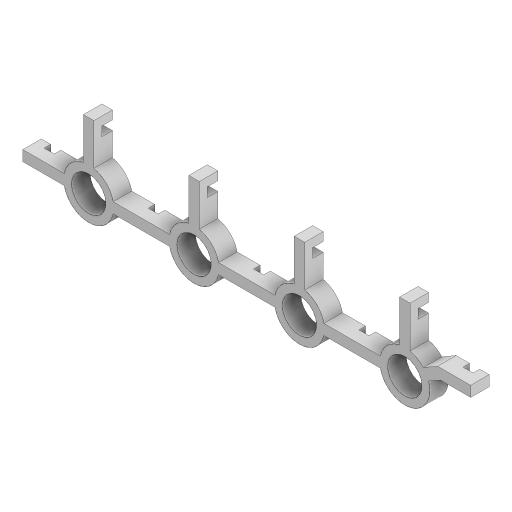
# Autodesk Inventor part: smic_jig_2
Saved by Autodesk Inventor 2024 (Build 280153000, 153)
## iProperties
Created: 2024-04-26
Part Number: smic_jig_2
Material: 一般
Document SubType Name: Modeling
Designer: TEA
Density: 1 g/cm^3
Appearance: 預設
Author: TEA
Autodesk Inventor part; units mm, degrees
ref_plane "YZ Plane" through (0, 0, 0) normal (1, 0, 0) x (0, 1, 0)
ref_plane "XZ Plane" through (0, 0, 0) normal (0, 1, 0) x (-1, 0, 0)
ref_plane "XY Plane" through (0, 0, 0) normal (0, 0, 1) x (1, 0, 0)
sketch "草圖1" plane through (0, 0, 0) normal (0, 0, 1) x (1, 0, 0)
  circle A0 centre (0, 0) radius 6.5
  circle A1 centre (0, 0) radius 9.5
  line L0 (0, 0) -> (16.7794, 0)
  circle A2 centre (40, 0) radius 6.5
  circle A3 centre (40, 0) radius 9.5
  circle A4 centre (80, 0) radius 6.5
  circle A5 centre (80, 0) radius 9.5
  circle A6 centre (120, 0) radius 6.5
  circle A7 centre (120, 0) radius 9.5
  line L1 (-25, 2) -> (128, 2)
  line L2 (128, 2) -> (128, -2)
  line L3 (128, -2) -> (-25, -2)
  line L4 (-25, -2) -> (-25, 2)
  line L5 (-2, 0) -> (2, 0)
  line L6 (2, 0) -> (2, 25)
  line L7 (2, 25) -> (-2, 25)
  line L8 (-2, 25) -> (-2, 0)
  line L9 (42, 0) -> (42, 25)
  line L10 (38, 0) -> (42, 0)
  line L11 (42, 25) -> (38, 25)
  line L12 (38, 25) -> (38, 0)
  line L13 (82, 0) -> (82, 25)
  line L14 (78, 0) -> (82, 0)
  line L15 (82, 25) -> (78, 25)
  line L16 (78, 25) -> (78, 0)
  line L17 (122, 0) -> (122, 25)
  line L18 (118, 0) -> (122, 0)
  line L19 (122, 25) -> (118, 25)
  line L20 (118, 25) -> (118, 0)
  line L21 (0, 0) -> (-12.3433, -7.1264)
  line L22 (0, 0) -> (14.2529, 0) construction
  line L23 (-12.4545, -9.5) -> (-25, -9.5)
  line L24 (-25, -9.5) -> (-25, -5.5)
  line L25 (-0.5359, 2) -> (14.2529, 2)
  line L26 (-12.4545, -9.5) -> (-7.0429, -6.3756)
  line L27 (0.5359, -2) -> (14.2529, -2)
  line L28 (-13.5263, -5.5) -> (-9.0429, -2.9115)
  line L29 (-25, -5.5) -> (-13.5263, -5.5)
  line L30 (-12.4545, 9.5) -> (-25, 9.5)
  line L31 (-25, 9.5) -> (-25, 5.5)
  line L32 (-12.4545, 9.5) -> (-7.0429, 6.3756)
  line L33 (-13.5263, 5.5) -> (-9.0429, 2.9115)
  line L34 (-25, 5.5) -> (-13.5263, 5.5)
  line L35 (42, 25) -> (78, 25)
  line L36 (60, 25) -> (60, 20)
  line L37 (132.4545, 9.5) -> (145, 9.5)
  line L38 (145, 9.5) -> (145, 5.5)
  line L39 (145, 5.5) -> (133.5263, 5.5)
  line L40 (133.5263, 5.5) -> (129.0429, 2.9115)
  line L41 (132.4545, 9.5) -> (127.0429, 6.3756)
  point P0 (-9.2871, -2)
  point P1 (-9.2871, 2)
  point P2 (30.7129, -2)
  point P3 (49.2871, -2)
  point P4 (70.7129, -2)
  point P5 (89.2871, -2)
  point P6 (110.7129, -2)
  point P7 (129.2871, -2)
  point P8 (129.2871, 2)
  point P9 (110.7129, 2)
  point P10 (89.2871, 2)
  point P11 (70.7129, 2)
  point P12 (49.2871, 2)
  point P13 (30.7129, 2)
  point P14 (9.2871, 2)
  point P15 (9.2871, -2)
  point P16 (118, 9.2871)
  point P17 (122, 9.2871)
  point P18 (78, 9.2871)
  point P19 (82, 9.2871)
  point P20 (38, 9.2871)
  point P21 (42, 9.2871)
  point P22 (-2, 9.2871)
  point P23 (2, 9.2871)
  point P24 (86.1847, -2)
  point P25 (113.8153, -2)
  point P26 (113.8153, 2)
  point P27 (86.1847, 2)
  point P28 (33.8153, -2)
  point P29 (33.8153, 2)
  point P30 (46.1847, -2)
  point P31 (73.8153, -2)
  point P32 (73.8153, 2)
  point P33 (46.1847, 2)
  point P34 (126.1847, 2)
  point P35 (126.1847, -2)
  dimension "d0" = 13
  dimension "d2" = 19
  dimension "d13" = 40
  dimension "d18" = 4
  dimension "d19" = 2
  dimension "d20" = 8
  dimension "d21" = 25
  dimension "d43" = 4
  dimension "d44" = 2
  dimension "d45" = 25
  dimension "d49" = 40
  dimension "d69" = 150
  dimension "d74" = 2
  dimension "d75" = 4
  dimension "d76" = 25
  dimension "d81" = 5
  constraints: 84 end point, 12 symmetric about line, 11 coincident, 8 centre point, 8 horizontal, 6 parallel, 5 midpoint, 3 perpendicular, 2 point on circle, 1 equal length, 1 tangent, 1 vertical, 45 other
  measures "d0" diameter of A0
  measures "d2" diameter of A1
  measures "d13" distance of A0.centre A2.centre
  measures "d18" distance of L1.end L2.end
  measures "d19" distance from line of point (0, 0) L1
  measures "d20" distance from line of A6.centre L2
  measures "d21" distance from line of point (0, 0) L4
  measures "d43" distance of L7.end L6.end
  measures "d44" distance from line of point (0, 0) L6
  measures "d45" distance of L7.end L5.start
  measures "d49" distance of L5.end L9.start
  measures "d69" angle of L21 L22
  measures "d74" distance between parallel lines of L21 L26
  measures "d75" distance of L23.end L24.end
  measures "d76" distance from line of A0.centre L24
  measures "d81" distance of L36.start L36.end
extrude "擠出1" add sketch "草圖1" along normal blind 7 contours L0 A1 L3 A0 | A0 L1 A1 L0 | A0 L6 A1 L1 | L3 A1 L21 A0 | A1 L1 A3 L3 | A0 L8 A1 L6 | L21 A1 L3 A0 | A0 L1 A1 L8 | A1 L8 L7 L6 | L3 A1 L1 A0 | L1 A2 L3 A3 | A3 L12 A2 L1 | L3 L4 L1 A1 | L3 A2 A3 | L12 L11 L9 A3 | A3 L9 A2 L12 | L3 A2 L1 A3 | A3 L1 A5 L3 | A3 L1 A2 L9 | L3 A4 A5 | A5 L1 A4 L3 | A5 L16 A4 L1 | L3 A4 L1 A5 | A5 L1 A7 L3 | L16 L15 L13 A5 | A5 L13 A4 L16 | L3 A6 L2 L1 L17 A7 | A7 L1 A6 L3 | A5 L1 A4 L13 | A7 L20 A6 L1 | L20 L19 L17 A7 | A7 L17 A6 L20 | A7 L41 L37 L38 L39 L40 | A6 L1 L2 L3
sketch "草圖3" plane through (49.2871, -2, 0) normal (0, -1, 0) x (1, 0, 0)
  line L0 (-31.1871, 0) -> (-27.3871, 0)
  line L1 (-27.3871, 0) -> (-27.3871, 2.5)
  line L2 (-27.3871, 2.5) -> (-31.1871, 2.5)
  line L3 (-31.1871, 2.5) -> (-31.1871, 0)
  line L4 (-31.1871, 0) -> (-27.3871, 2.5) construction
  line L5 (-27.3871, 0) -> (-31.1871, 2.5) construction
  line L6 (-18.5742, 0) -> (-18.5742, 7) projected
  line L7 (-40, 0) -> (-18.5742, 0) projected
  line L8 (-40, 0) -> (-18.5742, 0)
  line L9 (-29.2871, 0) -> (-29.2871, 1.25)
  line L10 (-70.6871, 0) -> (-66.8871, 0)
  line L11 (-66.8871, 0) -> (-66.8871, 2.5)
  line L12 (-66.8871, 2.5) -> (-70.6871, 2.5)
  line L13 (-70.6871, 2.5) -> (-70.6871, 0)
  line L14 (-70.6871, 0) -> (-66.8871, 2.5) construction
  line L15 (-66.8871, 0) -> (-70.6871, 2.5) construction
  line L16 (-68.7871, 0) -> (-68.7871, 1.25)
  line L17 (8.8129, 2.5) -> (8.8129, 0)
  line L18 (10.7129, 0) -> (10.7129, 1.25)
  line L19 (8.8129, 0) -> (12.6129, 0)
  line L20 (12.6129, 0) -> (12.6129, 2.5)
  line L21 (12.6129, 2.5) -> (8.8129, 2.5)
  line L22 (8.8129, 0) -> (12.6129, 2.5) construction
  line L23 (0, 0) -> (21.4258, 0)
  line L24 (12.6129, 0) -> (8.8129, 2.5) construction
  line L25 (48.8129, 2.5) -> (48.8129, 0)
  line L26 (50.7129, 0) -> (50.7129, 1.25)
  line L27 (48.8129, 0) -> (52.6129, 0)
  line L28 (52.6129, 0) -> (52.6129, 2.5)
  line L29 (52.6129, 2.5) -> (48.8129, 2.5)
  line L30 (48.8129, 0) -> (52.6129, 2.5) construction
  line L31 (40, 0) -> (61.4258, 0)
  line L32 (52.6129, 0) -> (48.8129, 2.5) construction
  line L33 (88.3129, 2.5) -> (88.3129, 0)
  line L34 (90.2129, 0) -> (90.2129, 1.25)
  line L35 (92.1129, 0) -> (92.1129, 2.5)
  line L36 (92.1129, 2.5) -> (88.3129, 2.5)
  line L37 (88.3129, 0) -> (92.1129, 2.5) construction
  line L38 (92.1129, 0) -> (88.3129, 2.5) construction
  line L39 (88.3129, 0) -> (92.1129, 0)
  line L40 (79.5, 0) -> (100.9258, 0)
  point P0 (-49.2871, 0)
  dimension "d22" = 3.8
  dimension "d23" = 2.5
  dimension "d25" = 1.25
  dimension "d35" = 39.5
  dimension "d54" = 20
  dimension "d101" = 40
  dimension "d108" = 39.5
  constraints: 78 end point, 6 midpoint, 4 horizontal, 3 equal length, 2 perpendicular, 1 collinear, 60 other
  measures "d22" distance of L2.end L1.end
  measures "d23" distance of L0.end L1.end
  measures "d25" distance of L9.start L9.end
  measures "d35" distance of L0.start L10.start
  measures "d54" distance of L9.start point (-49.287, 0)
  measures "d101" distance of L0.start L17.end
  measures "d108" distance of L25.end L33.end
extrude "擠出3" cut sketch "草圖3" along normal through all both and the other way through all
sketch "草圖4" plane through (-2, 9.2871, 0) normal (-1, 0, 0) x (0, 0, 1)
  line L0 (4, 8.9629) -> (0, 8.9629)
  line L1 (0, 8.9629) -> (0, 12.4629)
  line L2 (0, 12.4629) -> (4, 12.4629)
  line L3 (4, 12.4629) -> (4, 8.9629)
  line L4 (4, 8.9629) -> (0, 12.4629) construction
  line L5 (0, 8.9629) -> (4, 12.4629) construction
  line L6 (2, 10.7129) -> (0, 10.7129)
  line L7 (0, 0) -> (0, 15.7129) projected
  line L8 (0, -11.2871) -> (7, -11.2871) projected
  point P0 (0, 10.7129)
  dimension "d55" = 4
  dimension "d56" = 3.5
  dimension "d57" = 2
  dimension "d68" = 22
  constraints: 14 end point, 3 midpoint, 2 horizontal, 2 parallel, 1 perpendicular, 1 point on line
  measures "d55" distance of L1.end L2.end
  measures "d56" distance of L0.end L1.end
  measures "d57" distance of L6.start L6.end
  measures "d68" distance between parallel lines of L8 L6
extrude "擠出4" cut sketch "草圖4" against normal blind 10
sketch "草圖5" plane through (38, 9.2871, 0) normal (-1, 0, 0) x (0, 0, 1)
  line L0 (4, 12.4629) -> (4, 8.9629) projected
  line L1 (0, 12.4629) -> (4, 12.4629) projected
  line L2 (4, 8.9629) -> (0, 8.9629) projected
  line L3 (0, 15.7129) -> (0, 0) projected
  point P0 (0, -9.2871)
extrude "擠出5" cut sketch "草圖5" against normal blind 10
sketch "草圖6" plane through (78, 9.2871, 0) normal (-1, 0, 0) x (0, 0, 1)
  line L0 (4, 12.4629) -> (4, 8.9629) projected
  line L1 (0, 12.4629) -> (4, 12.4629) projected
  line L2 (4, 8.9629) -> (0, 8.9629) projected
  line L3 (0, 15.7129) -> (0, 0) projected
  point P0 (0, -9.2871)
extrude "擠出6" cut sketch "草圖6" against normal blind 10
sketch "草圖7" plane through (118, 9.2871, 0) normal (-1, 0, 0) x (0, 0, 1)
  line L0 (4, 12.4629) -> (4, 8.9629) projected
  line L1 (0, 12.4629) -> (4, 12.4629) projected
  line L2 (4, 8.9629) -> (0, 8.9629) projected
  line L3 (0, 15.7129) -> (0, 0) projected
  point P0 (0, -9.2871)
extrude "擠出7" cut sketch "草圖7" against normal blind 10
